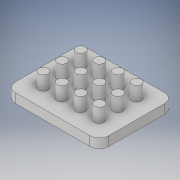
# Autodesk Inventor part: 練習二
Saved by Autodesk Inventor 2017 (Build 210142000, 142)
## iProperties
Part Number: 練習二
Material: 一般
Document SubType Name: Modeling
Designer: user
Density: 1 g/cm^3
Appearance: 預設
Author: user
Autodesk Inventor part; units mm, degrees
ref_plane "YZ Plane" through (0, 0, 0) normal (1, 0, 0) x (0, 1, 0)
ref_plane "XZ Plane" through (0, 0, 0) normal (0, 1, 0) x (-1, 0, 0)
ref_plane "XY Plane" through (0, 0, 0) normal (0, 0, 1) x (1, 0, 0)
sketch "草圖1" plane through (0, 0, 0) normal (0, 1, 0) x (-1, 0, 0)
  line L0 (-10, 0) -> (-90, 0)
  line L1 (-100, -10) -> (-100, -70)
  line L2 (-90, -80) -> (-10, -80)
  line L3 (0, -70) -> (0, -10)
  arc A0 (-90, 0) -> (-100, -10) centre (-90, -10) ccw
  arc A1 (-100, -70) -> (-90, -80) centre (-90, -70) ccw
  arc A2 (-10, -80) -> (0, -70) centre (-10, -70) ccw
  arc A3 (0, -10) -> (-10, 0) centre (-10, -10) ccw
  point P0 (0, 0)
  point P1 (-100, 0)
  point P2 (0, -80)
  dimension "d0" = 100
  dimension "d1" = 80
  dimension "d2" = 10
  constraints: 8 end point, 8 point on circle, 8 tangent, 6 point on line, 4 centre point, 3 equal radius, 2 parallel, 1 horizontal, 1 perpendicular
  measures "d0" distance of point (0, 0) point (-100, 0)
  measures "d1" distance of point (0, -80) point (0, 0)
  measures "d2" radius of A0
extrude "擠出1" add sketch "草圖1" along normal blind 10
sketch "草圖2" plane through (0, 10, 0) normal (0, 1, 0) x (1, 0, 0)
  circle A0 centre (80, 20) radius 5
  line L0 (100, 10) -> (100, 70) projected
  line L1 (10, 0) -> (90, 0) projected
  point P0 (0, 0)
  dimension "d5" = 20
  dimension "d6" = 20
  dimension "d7" = 10
  constraints: 1 centre point
  measures "d5" distance from line of L0 A0.centre
  measures "d6" distance from line of A0.centre L1
  measures "d7" diameter of A0
extrude "擠出2" add sketch "草圖2" along normal blind 15
pattern_linear "矩形陣列1" count 4 spacing 20 along (-1, 0, 0) count 3 spacing 20 along (0, 0, -1) of "擠出2"
